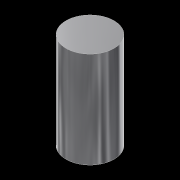
# Autodesk Inventor part: Part3
Saved by Autodesk Inventor 2021.1 (Build 251245000, 245)
## iProperties
Created: 2020-09-01
Part Number: Part3
Material: A5052
Document SubType Name: Modeling
Designer: Hashimoto
Mass: 4.25753 g
Surface Area: 7.85398 cm^2
Volume: 1.5708 cm^3
Density: 2.71043 g/cm^3
Appearance: アルミニウム - つや出し
Author: Hashimoto
Autodesk Inventor part; units mm, degrees
ref_plane "YZ Plane" through (0, 0, 0) normal (1, 0, 0) x (0, 1, 0)
ref_plane "XZ Plane" through (0, 0, 0) normal (0, 1, 0) x (-1, 0, 0)
ref_plane "XY Plane" through (0, 0, 0) normal (0, 0, 1) x (1, 0, 0)
sketch "スケッチ22" plane through (0, 0, 0) normal (0, 0, 1) x (1, 0, 0)
  circle A0 centre (0, 0) radius 5
  dimension "d137" = 10
  constraints: 1 centre point, 1 coincident
  measures "d137" diameter of A0
extrude "押し出し14" add sketch "スケッチ22" along normal blind 20
